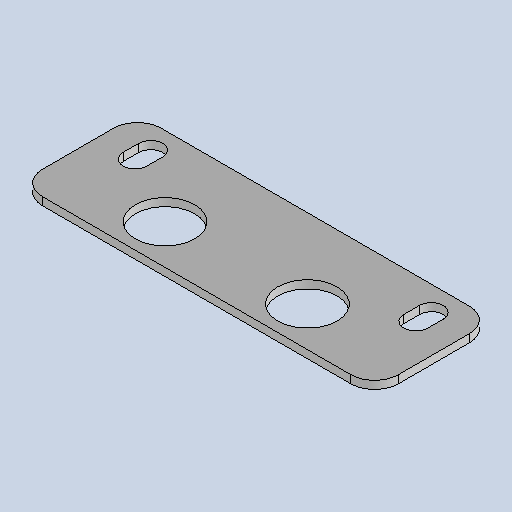
# Autodesk Inventor part: motor pillar 4
Saved by Autodesk Inventor 2025.3 (Build 293356030, 356C)
## iProperties
Created: 2025-09-03
Part Number: motor pillar 4
Material: Generic
Document SubType Name: Sheet Metal
Designer: admin
Density: 1 g/cm^3
Sheet Metal Rule: Default
Appearance: Default
Mass: 4.42224 g
Surface Area: 51.7753 cm^2
Volume: 4.42224 cm^3
Flat Pattern Width: 3 cm
Flat Pattern Length: 9 cm
Flat Pattern Area: 27 cm^2
Sheet Metal Width: 30,000 mm
Sheet Metal Length: 90,000 mm
Sheet Metal Area: 2700,000 mm^2
Author: admin
Autodesk Inventor part; units mm, degrees
ref_plane "YZ Plane" through (0, 0, 0) normal (1, 0, 0) x (0, 1, 0)
ref_plane "XZ Plane" through (0, 0, 0) normal (0, 1, 0) x (-1, 0, 0)
ref_plane "XY Plane" through (0, 0, 0) normal (0, 0, 1) x (1, 0, 0)
sketch "Sketch1" plane through (0, 0, 0) normal (0, 0, 1) x (1, 0, 0)
  line L0 (-45, 15) -> (45, 15)
  line L1 (45, 15) -> (45, -15)
  line L2 (45, -15) -> (-45, -15)
  line L3 (-45, -15) -> (-45, 15)
  line L4 (-45, 15) -> (45, -15) construction
  line L5 (45, 15) -> (-45, -15) construction
  circle A0 centre (18, -5) radius 7.5
  circle A1 centre (-18, -5) radius 7.5
  line L6 (0, 15) -> (0, -15) construction
  line L7 (25.5, -5) -> (25.5, -15)
  line L8 (10.5, -5) -> (10.5, -15)
  line L9 (-10.5, -5) -> (-10.5, -15)
  line L10 (-25.5, -5) -> (-25.5, -15)
  line L11 (35.5, 8.8807) -> (35.5, 4.8807) construction
  line L12 (38.5, 8.8807) -> (38.5, 4.8807)
  line L13 (32.5, 4.8807) -> (32.5, 8.8807)
  arc A2 (38.5, 8.8807) -> (32.5, 8.8807) centre (35.5, 8.8807) ccw
  arc A3 (32.5, 4.8807) -> (38.5, 4.8807) centre (35.5, 4.8807) ccw
  line L14 (-35.5, 8.8807) -> (-35.5, 4.8807) construction
  line L15 (-38.5, 8.8807) -> (-38.5, 4.8807)
  line L16 (-32.5, 4.8807) -> (-32.5, 8.8807)
  arc A4 (-32.5, 8.8807) -> (-38.5, 8.8807) centre (-35.5, 8.8807) ccw
  arc A5 (-38.5, 4.8807) -> (-32.5, 4.8807) centre (-35.5, 4.8807) ccw
  point P0 (0, 0)
  point P1 (0, 0)
  point P2 (35.5, 6.8807)
  point P3 (-35.5, 6.8807)
  dimension "d0" = 90
  dimension "d1" = 30
  dimension "d2" = 15
  dimension "d3" = 36
  dimension "d6" = 10
  dimension "d7" = 6
  dimension "d8" = 4
  dimension "d9" = 71
  measures "d0" distance of L1.end L2.end
  measures "d1" distance of L0.end L1.end
  measures "d2" diameter of A1
  measures "d3" distance of A0.centre A1.centre
  measures "d6" distance from line of L2 A0.centre
  measures "d7" distance between parallel lines of L13 L12
  measures "d8" distance of L11.start L11.end
  measures "d9" distance between parallel lines of L14 L11
extrude "Plate1" add sketch "Sketch1" along normal blind 2 contours L0 L1 L2 L7 A0 L8 L9 A1 L10 L3 | L10 A1 L9 L2 | L2 L8 A0 L7
fillet "Corner Round1" radius 6 4 edges at (-45, 15, 1) (-45, -15, 1) (45, 15, 1) (45, -15, 1)
equation "\"d4\" = Thickness"
equation "\"BendRadius\" = Thickness"
equation "\"BendReliefWidth\" = Thickness"
equation "\"BendReliefDepth\" = 0.5 * Thickness"
equation "\"CornerReliefSize\" = 4 * Thickness"
equation "\"MinimumRemnant\" = 2 * Thickness"
equation "\"TransitionRadius\" = BendRadius"
equation "\"JacobiRadiusSize\" = BendRadius"
equation "\"GapSize\" = Thickness"
equation "\"Thickness\" = 2"
body "Solid1"
